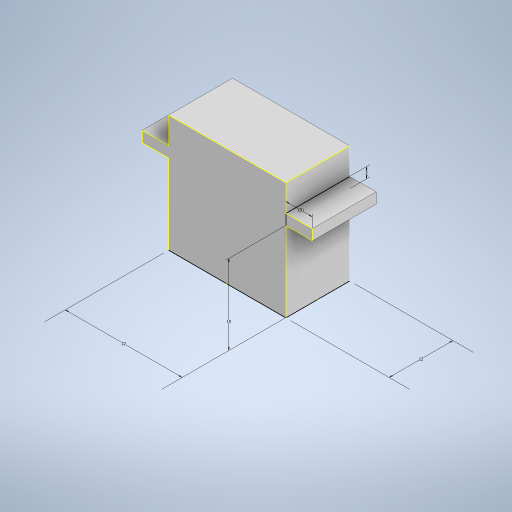
# Autodesk Inventor part: 서보모터
Saved by Autodesk Inventor 2023 (Build 270158000, 158)
## iProperties
Created: 2023-08-25
Part Number: 서보모터
Material: 일반
Document SubType Name: Modeling
Designer: rlatk
Density: 1 g/cm^3
Appearance: 기본값
Author: rlatk
Autodesk Inventor part; units mm, degrees
ref_plane "YZ Plane" through (0, 0, 0) normal (1, 0, 0) x (0, 1, 0)
ref_plane "XZ Plane" through (0, 0, 0) normal (0, 1, 0) x (-1, 0, 0)
ref_plane "XY Plane" through (0, 0, 0) normal (0, 0, 1) x (1, 0, 0)
sketch "스케치1" plane through (0, 0, 0) normal (0, 1, 0) x (-1, 0, 0)
  line L0 (11, -6) -> (-11, -6)
  line L1 (-11, -6) -> (-11, 6)
  line L2 (-11, 6) -> (11, 6)
  line L3 (11, 6) -> (11, -6)
  line L4 (11, -6) -> (-11, 6) construction
  line L5 (-11, -6) -> (11, 6) construction
  point P0 (0, 0)
  dimension "d0" = 22
  dimension "d1" = 12
  constraints: 12 end point, 2 midpoint, 2 parallel, 1 horizontal, 1 perpendicular
  measures "d0" distance of L1.end L2.end
  measures "d1" distance of L0.end L1.end
extrude "돌출1" add sketch "스케치1" along normal blind 22
sketch "스케치2" plane through (11, 0, 6) normal (1, 0, 0) x (0, 0, -1)
  line L0 (0, 0) -> (12, 0) projected
  line L1 (12, 0) -> (12, 22) projected
  line L2 (0, 22) -> (12, 22) projected
  line L3 (0, 0) -> (0, 22) projected
  line L4 (0, 17) -> (12, 17)
  line L5 (12, 17) -> (12, 15)
  line L6 (12, 15) -> (0, 15)
  line L7 (0, 15) -> (0, 17)
  point P0 (6, 0)
  point P1 (0, 15)
  dimension "d4" = 2
  dimension "d5" = 15
  constraints: 8 end point, 2 parallel, 2 point on line, 1 horizontal, 1 perpendicular
  measures "d4" distance of L4.end L5.end
  measures "d5" distance between parallel lines of L0 L6
extrude "돌출2" add sketch "스케치2" along normal blind 5 contours L3 L4 L1 L6
mirror "미러1" about plane through (0, 0, 0) normal (1, 0, 0) of "돌출2"
sketch "스케치3" plane through (-11, 0, 6) normal (0, 0, 1) x (1, 0, 0)
  line L0 (0, 0) -> (22, 0) projected
  line L1 (22, 0) -> (22, 15) projected
  line L2 (22, 15) -> (27, 15) projected
  line L3 (27, 17) -> (27, 15) projected
  line L4 (22, 17) -> (27, 17) projected
  line L5 (22, 17) -> (22, 22) projected
  line L6 (0, 22) -> (22, 22) projected
  line L7 (0, 17) -> (0, 22) projected
  line L8 (0, 17) -> (-5, 17) projected
  line L9 (-5, 17) -> (-5, 15) projected
  line L10 (0, 15) -> (-5, 15) projected
  line L11 (0, 0) -> (0, 15) projected
  point P0 (11, 0)
  dimension "d8" = 5
  measures "d8" distance between parallel lines of L5 L3
